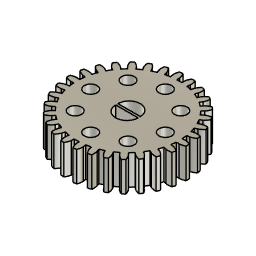
Shaft Arm Joint 0-1 Gear (Autodesk Fusion 360 design; units mm, degrees)
Autodesk Fusion 360 part; units mm, degrees
note: some values were not read from the file. Set by a fixed rule: which sketch regions a step uses.
(part 1 of 20)
sketch "スケッチ1" plane through (0, 0, 0) normal (0, 0, 1) x (1, 0, 0) in component "Component"
  spline S0 degree 5 poles (14.4985, -0.8405) (14.4986, -0.8405) (14.4987, -0.8405) (14.499, -0.8405) (14.4993, -0.8405) (14.4999, -0.8405) (14.5005, -0.8406) (14.5012, -0.8406) (14.502, -0.8406) (14.5028, -0.8406) (14.5037, -0.8407) (14.5048, -0.8407) (14.5058, -0.8407) (14.507, -0.8407) (14.5082, -0.8408) (14.5096, -0.8408) (14.5109, -0.8408) (14.5124, -0.8408) (14.5139, -0.8409) (14.5155, -0.8409) (14.5172, -0.8409) (14.519, -0.8409) (14.5208, -0.8409) (14.5226, -0.8409) (14.5246, -0.8409) (14.5266, -0.8409) (14.5287, -0.8409) (14.5309, -0.8409) (14.5331, -0.8408) (14.5354, -0.8408) (14.5377, -0.8408) (14.5401, -0.8407) (14.5426, -0.8407) (14.5452, -0.8406) (14.5478, -0.8406) (14.5504, -0.8405) (14.5532, -0.8404) (14.556, -0.8403) (14.5588, -0.8402) (14.5617, -0.8401) (14.5647, -0.84) (14.5677, -0.8399) (14.5708, -0.8398) (14.574, -0.8396) (14.5772, -0.8395) (14.5805, -0.8393) (14.5838, -0.8392) (14.5872, -0.839) (14.5906, -0.8388) (14.5941, -0.8386) (14.5977, -0.8384) (14.6013, -0.8382) (14.605, -0.838) (14.6087, -0.8377) (14.6124, -0.8375) (14.6163, -0.8372) (14.6202, -0.8369) (14.6241, -0.8366) (14.6281, -0.8363) (14.6321, -0.836) (14.6362, -0.8357) (14.6404, -0.8354) (14.6446, -0.835) (14.6488, -0.8347) (14.6531, -0.8343) (14.6574, -0.8339) (14.6618, -0.8335) (14.6663, -0.8331) (14.6708, -0.8326) (14.6753, -0.8322) (14.6799, -0.8317) (14.6846, -0.8313) (14.6893, -0.8308) (14.694, -0.8303) (14.6988, -0.8298) (14.7036, -0.8292) (14.7085, -0.8287) (14.7134, -0.8281) (14.7184, -0.8275) (14.7234, -0.8269) (14.7285, -0.8263) (14.7336, -0.8257) (14.7387, -0.8251) (14.7439, -0.8244) (14.7492, -0.8237) (14.7545, -0.8231) (14.7598, -0.8224) (14.7652, -0.8216) (14.7706, -0.8209) (14.7761, -0.8201) (14.7816, -0.8194) (14.7871, -0.8186) (14.7927, -0.8178) (14.7983, -0.817) (14.804, -0.8161) (14.8097, -0.8153) (14.8155, -0.8144) (14.8213, -0.8135) (14.8271, -0.8126) (14.833, -0.8117) (14.8389, -0.8107) (14.8449, -0.8097) (14.8509, -0.8088) (14.8569, -0.8078) (14.863, -0.8067) (14.8691, -0.8057) (14.8753, -0.8047) (14.8814, -0.8036) (14.8877, -0.8025) (14.8939, -0.8014) (14.9003, -0.8002) (14.9066, -0.7991) (14.913, -0.7979) (14.9194, -0.7967) (14.9259, -0.7955) (14.9324, -0.7943) (14.9389, -0.7931) (14.9455, -0.7918) (14.9521, -0.7905) (14.9587, -0.7892) (14.9654, -0.7879) (14.9721, -0.7865) (14.9788, -0.7852) (14.9856, -0.7838) (14.9924, -0.7824) (14.9993, -0.781) (15.0062, -0.7795) (15.0131, -0.778) (15.02, -0.7766) (15.027, -0.775) (15.0341, -0.7735) (15.0411, -0.772) (15.0482, -0.7704) (15.0553, -0.7688) (15.0625, -0.7672) (15.0697, -0.7656) (15.0769, -0.7639) (15.0841, -0.7622) (15.0914, -0.7605) (15.0987, -0.7588) (15.1061, -0.7571) (15.1135, -0.7553) (15.1209, -0.7535) (15.1283, -0.7517) (15.1358, -0.7499) (15.1433, -0.7481) (15.1508, -0.7462) (15.1584, -0.7443) (15.166, -0.7424) (15.1736, -0.7405) (15.1813, -0.7385) (15.1889, -0.7365) (15.1967, -0.7345) (15.2044, -0.7325) (15.2122, -0.7305) (15.22, -0.7284) (15.2278, -0.7263) (15.2357, -0.7242) (15.2436, -0.7221) (15.2515, -0.7199) (15.2594, -0.7177) (15.2674, -0.7155) (15.2754, -0.7133) (15.2834, -0.7111) (15.2915, -0.7088) (15.2996, -0.7065) (15.3077, -0.7042) (15.3158, -0.7018) (15.324, -0.6995) (15.3322, -0.6971) (15.3404, -0.6947) (15.3487, -0.6923) (15.3569, -0.6898) (15.3652, -0.6873) (15.3736, -0.6848) (15.3819, -0.6823) (15.3903, -0.6797) (15.3987, -0.6772) (15.4071, -0.6746) (15.4156, -0.672) (15.4241, -0.6693) (15.4326, -0.6667) (15.4411, -0.664) (15.4497, -0.6613) (15.4582, -0.6585) (15.4668, -0.6558) (15.4755, -0.653) (15.4841, -0.6502) (15.4928, -0.6473) (15.5015, -0.6445) (15.5102, -0.6416) (15.519, -0.6387) (15.5278, -0.6358) (15.5365, -0.6328) (15.5454, -0.6298) (15.5542, -0.6268) (15.5631, -0.6238) (15.572, -0.6207) (15.5809, -0.6177) (15.5898, -0.6146) (15.5988, -0.6114) (15.6077, -0.6083) (15.6167, -0.6051) (15.6258, -0.6019) (15.6348, -0.5987) (15.6439, -0.5955) (15.653, -0.5922) (15.6621, -0.5889) (15.6712, -0.5856) (15.6803, -0.5822) (15.6895, -0.5789) (15.6987, -0.5755) (15.7079, -0.572) (15.7172, -0.5686) (15.7264, -0.5651) (15.7357, -0.5616) (15.745, -0.5581) (15.7543, -0.5546) (15.7636, -0.551) (15.773, -0.5474) (15.7824, -0.5438) (15.7918, -0.5401) (15.8012, -0.5365) (15.8106, -0.5328) (15.8201, -0.529) (15.8295, -0.5253) (15.839, -0.5215) (15.8486, -0.5177) (15.8581, -0.5139) (15.8676, -0.5101) (15.8772, -0.5062) (15.8868, -0.5023) (15.8964, -0.4984) (15.906, -0.4944) (15.9157, -0.4904) (15.9253, -0.4864) (15.935, -0.4824) (15.9447, -0.4784) (15.9544, -0.4743) (15.9641, -0.4702) (15.9739, -0.466) (15.9817, -0.4627) (15.9876, -0.4602) (15.9915, -0.4585) (15.9935, -0.4577) knots 0 0 0 0 0 0 0.00416667 0.00833333 0.0125 0.01666667 0.02083333 0.025 0.02916667 0.03333333 0.0375 0.04166667 0.04583333 0.05 0.05416667 0.05833333 0.0625 0.06666667 0.07083333 0.075 0.07916667 0.08333333 0.0875 0.09166667 0.09583333 0.1 0.10416667 0.10833333 0.1125 0.11666667 0.12083333 0.125 0.12916667 0.13333333 0.1375 0.14166667 0.14583333 0.15 0.15416667 0.15833333 0.1625 0.16666667 0.17083333 0.175 0.17916667 0.18333333 0.1875 0.19166667 0.19583333 0.2 0.20416667 0.20833333 0.2125 0.21666667 0.22083333 0.225 0.22916667 0.23333333 0.2375 0.24166667 0.24583333 0.25 0.25416667 0.25833333 0.2625 0.26666667 0.27083333 0.275 0.27916667 0.28333333 0.2875 0.29166667 0.29583333 0.3 0.30416667 0.30833333 0.3125 0.31666667 0.32083333 0.325 0.32916667 0.33333333 0.3375 0.34166667 0.34583333 0.35 0.35416667 0.35833333 0.3625 0.36666667 0.37083333 0.375 0.37916667 0.38333333 0.3875 0.39166667 0.39583333 0.4 0.40416667 0.40833333 0.4125 0.41666667 0.42083333 0.425 0.42916667 0.43333333 0.4375 0.44166667 0.44583333 0.45 0.45416667 0.45833333 0.4625 0.46666667 0.47083333 0.475 0.47916667 0.48333333 0.4875 0.49166667 0.49583333 0.5 0.50416667 0.50833333 0.5125 0.51666667 0.52083333 0.525 0.52916667 0.53333333 0.5375 0.54166667 0.54583333 0.55 0.55416667 0.55833333 0.5625 0.56666667 0.57083333 0.575 0.57916667 0.58333333 0.5875 0.59166667 0.59583333 0.6 0.60416667 0.60833333 0.6125 0.61666667 0.62083333 0.625 0.62916667 0.63333333 0.6375 0.64166667 0.64583333 0.65 0.65416667 0.65833333 0.6625 0.66666667 0.67083333 0.675 0.67916667 0.68333333 0.6875 0.69166667 0.69583333 0.7 0.70416667 0.70833333 0.7125 0.71666667 0.72083333 0.725 0.72916667 0.73333333 0.7375 0.74166667 0.74583333 0.75 0.75416667 0.75833333 0.7625 0.76666667 0.77083333 0.775 0.77916667 0.78333333 0.7875 0.79166667 0.79583333 0.8 0.80416667 0.80833333 0.8125 0.81666667 0.82083333 0.825 0.82916667 0.83333333 0.8375 0.84166667 0.84583333 0.85 0.85416667 0.85833333 0.8625 0.86666667 0.87083333 0.875 0.87916667 0.88333333 0.8875 0.89166667 0.89583333 0.9 0.90416667 0.90833333 0.9125 0.91666667 0.92083333 0.925 0.92916667 0.93333333 0.9375 0.94166667 0.94583333 0.95 0.95416667 0.95833333 0.9625 0.96666667 0.97083333 0.975 0.97916667 0.98333333 0.9875 0.99166667 0.99583333 1 1 1 1 1 1
  spline S1 degree 5 poles (14.4985, 0.8405) (14.4986, 0.8405) (14.4987, 0.8405) (14.499, 0.8405) (14.4993, 0.8405) (14.4999, 0.8405) (14.5005, 0.8406) (14.5012, 0.8406) (14.502, 0.8406) (14.5028, 0.8406) (14.5037, 0.8407) (14.5048, 0.8407) (14.5058, 0.8407) (14.507, 0.8407) (14.5082, 0.8408) (14.5096, 0.8408) (14.5109, 0.8408) (14.5124, 0.8408) (14.5139, 0.8409) (14.5155, 0.8409) (14.5172, 0.8409) (14.519, 0.8409) (14.5208, 0.8409) (14.5226, 0.8409) (14.5246, 0.8409) (14.5266, 0.8409) (14.5287, 0.8409) (14.5309, 0.8409) (14.5331, 0.8408) (14.5354, 0.8408) (14.5377, 0.8408) (14.5401, 0.8407) (14.5426, 0.8407) (14.5452, 0.8406) (14.5478, 0.8406) (14.5504, 0.8405) (14.5532, 0.8404) (14.556, 0.8403) (14.5588, 0.8402) (14.5617, 0.8401) (14.5647, 0.84) (14.5677, 0.8399) (14.5708, 0.8398) (14.574, 0.8396) (14.5772, 0.8395) (14.5805, 0.8393) (14.5838, 0.8392) (14.5872, 0.839) (14.5906, 0.8388) (14.5941, 0.8386) (14.5977, 0.8384) (14.6013, 0.8382) (14.605, 0.838) (14.6087, 0.8377) (14.6124, 0.8375) (14.6163, 0.8372) (14.6202, 0.8369) (14.6241, 0.8366) (14.6281, 0.8363) (14.6321, 0.836) (14.6362, 0.8357) (14.6404, 0.8354) (14.6446, 0.835) (14.6488, 0.8347) (14.6531, 0.8343) (14.6574, 0.8339) (14.6618, 0.8335) (14.6663, 0.8331) (14.6708, 0.8326) (14.6753, 0.8322) (14.6799, 0.8317) (14.6846, 0.8313) (14.6893, 0.8308) (14.694, 0.8303) (14.6988, 0.8298) (14.7036, 0.8292) (14.7085, 0.8287) (14.7134, 0.8281) (14.7184, 0.8275) (14.7234, 0.8269) (14.7285, 0.8263) (14.7336, 0.8257) (14.7387, 0.8251) (14.7439, 0.8244) (14.7492, 0.8237) (14.7545, 0.8231) (14.7598, 0.8224) (14.7652, 0.8216) (14.7706, 0.8209) (14.7761, 0.8201) (14.7816, 0.8194) (14.7871, 0.8186) (14.7927, 0.8178) (14.7983, 0.817) (14.804, 0.8161) (14.8097, 0.8153) (14.8155, 0.8144) (14.8213, 0.8135) (14.8271, 0.8126) (14.833, 0.8117) (14.8389, 0.8107) (14.8449, 0.8097) (14.8509, 0.8088) (14.8569, 0.8078) (14.863, 0.8067) (14.8691, 0.8057) (14.8753, 0.8047) (14.8814, 0.8036) (14.8877, 0.8025) (14.8939, 0.8014) (14.9003, 0.8002) (14.9066, 0.7991) (14.913, 0.7979) (14.9194, 0.7967) (14.9259, 0.7955) (14.9324, 0.7943) (14.9389, 0.7931) (14.9455, 0.7918) (14.9521, 0.7905) (14.9587, 0.7892) (14.9654, 0.7879) (14.9721, 0.7865) (14.9788, 0.7852) (14.9856, 0.7838) (14.9924, 0.7824) (14.9993, 0.781) (15.0062, 0.7795) (15.0131, 0.778) (15.02, 0.7766) (15.027, 0.775) (15.0341, 0.7735) (15.0411, 0.772) (15.0482, 0.7704) (15.0553, 0.7688) (15.0625, 0.7672) (15.0697, 0.7656) (15.0769, 0.7639) (15.0841, 0.7622) (15.0914, 0.7605) (15.0987, 0.7588) (15.1061, 0.7571) (15.1135, 0.7553) (15.1209, 0.7535) (15.1283, 0.7517) (15.1358, 0.7499) (15.1433, 0.7481) (15.1508, 0.7462) (15.1584, 0.7443) (15.166, 0.7424) (15.1736, 0.7405) (15.1813, 0.7385) (15.1889, 0.7365) (15.1967, 0.7345) (15.2044, 0.7325) (15.2122, 0.7305) (15.22, 0.7284) (15.2278, 0.7263) (15.2357, 0.7242) (15.2436, 0.7221) (15.2515, 0.7199) (15.2594, 0.7177) (15.2674, 0.7155) (15.2754, 0.7133) (15.2834, 0.7111) (15.2915, 0.7088) (15.2996, 0.7065) (15.3077, 0.7042) (15.3158, 0.7018) (15.324, 0.6995) (15.3322, 0.6971) (15.3404, 0.6947) (15.3487, 0.6923) (15.3569, 0.6898) (15.3652, 0.6873) (15.3736, 0.6848) (15.3819, 0.6823) (15.3903, 0.6797) (15.3987, 0.6772) (15.4071, 0.6746) (15.4156, 0.672) (15.4241, 0.6693) (15.4326, 0.6667) (15.4411, 0.664) (15.4497, 0.6613) (15.4582, 0.6585) (15.4668, 0.6558) (15.4755, 0.653) (15.4841, 0.6502) (15.4928, 0.6473) (15.5015, 0.6445) (15.5102, 0.6416) (15.519, 0.6387) (15.5278, 0.6358) (15.5365, 0.6328) (15.5454, 0.6298) (15.5542, 0.6268) (15.5631, 0.6238) (15.572, 0.6207) (15.5809, 0.6177) (15.5898, 0.6146) (15.5988, 0.6114) (15.6077, 0.6083) (15.6167, 0.6051) (15.6258, 0.6019) (15.6348, 0.5987) (15.6439, 0.5955) (15.653, 0.5922) (15.6621, 0.5889) (15.6712, 0.5856) (15.6803, 0.5822) (15.6895, 0.5789) (15.6987, 0.5755) (15.7079, 0.572) (15.7172, 0.5686) (15.7264, 0.5651) (15.7357, 0.5616) (15.745, 0.5581) (15.7543, 0.5546) (15.7636, 0.551) (15.773, 0.5474) (15.7824, 0.5438) (15.7918, 0.5401) (15.8012, 0.5365) (15.8106, 0.5328) (15.8201, 0.529) (15.8295, 0.5253) (15.839, 0.5215) (15.8486, 0.5177) (15.8581, 0.5139) (15.8676, 0.5101) (15.8772, 0.5062) (15.8868, 0.5023) (15.8964, 0.4984) (15.906, 0.4944) (15.9157, 0.4904) (15.9253, 0.4864) (15.935, 0.4824) (15.9447, 0.4784) (15.9544, 0.4743) (15.9641, 0.4702) (15.9739, 0.466) (15.9817, 0.4627) (15.9876, 0.4602) (15.9915, 0.4585) (15.9935, 0.4577) knots 0 0 0 0 0 0 0.00416667 0.00833333 0.0125 0.01666667 0.02083333 0.025 0.02916667 0.03333333 0.0375 0.04166667 0.04583333 0.05 0.05416667 0.05833333 0.0625 0.06666667 0.07083333 0.075 0.07916667 0.08333333 0.0875 0.09166667 0.09583333 0.1 0.10416667 0.10833333 0.1125 0.11666667 0.12083333 0.125 0.12916667 0.13333333 0.1375 0.14166667 0.14583333 0.15 0.15416667 0.15833333 0.1625 0.16666667 0.17083333 0.175 0.17916667 0.18333333 0.1875 0.19166667 0.19583333 0.2 0.20416667 0.20833333 0.2125 0.21666667 0.22083333 0.225 0.22916667 0.23333333 0.2375 0.24166667 0.24583333 0.25 0.25416667 0.25833333 0.2625 0.26666667 0.27083333 0.275 0.27916667 0.28333333 0.2875 0.29166667 0.29583333 0.3 0.30416667 0.30833333 0.3125 0.31666667 0.32083333 0.325 0.32916667 0.33333333 0.3375 0.34166667 0.34583333 0.35 0.35416667 0.35833333 0.3625 0.36666667 0.37083333 0.375 0.37916667 0.38333333 0.3875 0.39166667 0.39583333 0.4 0.40416667 0.40833333 0.4125 0.41666667 0.42083333 0.425 0.42916667 0.43333333 0.4375 0.44166667 0.44583333 0.45 0.45416667 0.45833333 0.4625 0.46666667 0.47083333 0.475 0.47916667 0.48333333 0.4875 0.49166667 0.49583333 0.5 0.50416667 0.50833333 0.5125 0.51666667 0.52083333 0.525 0.52916667 0.53333333 0.5375 0.54166667 0.54583333 0.55 0.55416667 0.55833333 0.5625 0.56666667 0.57083333 0.575 0.57916667 0.58333333 0.5875 0.59166667 0.59583333 0.6 0.60416667 0.60833333 0.6125 0.61666667 0.62083333 0.625 0.62916667 0.63333333 0.6375 0.64166667 0.64583333 0.65 0.65416667 0.65833333 0.6625 0.66666667 0.67083333 0.675 0.67916667 0.68333333 0.6875 0.69166667 0.69583333 0.7 0.70416667 0.70833333 0.7125 0.71666667 0.72083333 0.725 0.72916667 0.73333333 0.7375 0.74166667 0.74583333 0.75 0.75416667 0.75833333 0.7625 0.76666667 0.77083333 0.775 0.77916667 0.78333333 0.7875 0.79166667 0.79583333 0.8 0.80416667 0.80833333 0.8125 0.81666667 0.82083333 0.825 0.82916667 0.83333333 0.8375 0.84166667 0.84583333 0.85 0.85416667 0.85833333 0.8625 0.86666667 0.87083333 0.875 0.87916667 0.88333333 0.8875 0.89166667 0.89583333 0.9 0.90416667 0.90833333 0.9125 0.91666667 0.92083333 0.925 0.92916667 0.93333333 0.9375 0.94166667 0.94583333 0.95 0.95416667 0.95833333 0.9625 0.96666667 0.97083333 0.975 0.97916667 0.98333333 0.9875 0.99166667 0.99583333 1 1 1 1 1 1
  spline S2 degree 5 poles (14.4979, -0.8404) (14.4979, -0.8404) (14.498, -0.8404) (14.498, -0.8404) (14.4981, -0.8404) (14.4983, -0.8405) (14.4984, -0.8405) (14.4984, -0.8405) (14.4985, -0.8405) (14.4985, -0.8405) knots 0 0 0 0 0 0 0.2 0.4 0.6 0.8 1 1 1 1 1 1
  spline S3 degree 5 poles (14.4979, 0.8404) (14.4979, 0.8404) (14.498, 0.8404) (14.498, 0.8404) (14.4981, 0.8404) (14.4983, 0.8405) (14.4984, 0.8405) (14.4984, 0.8405) (14.4985, 0.8405) (14.4985, 0.8405) knots 0 0 0 0 0 0 0.2 0.4 0.6 0.8 1 1 1 1 1 1
  line L0 (0, 0) -> (14.4979, -0.8404)
  line L1 (0, 0) -> (14.4979, 0.8404)
  arc A0 (15.9935, -0.4577) -> (15.9935, 0.4577) centre (0, 0) ccw
  point P0 (14.5005, -0.8406)
  point P1 (14.5037, -0.8407)
  point P2 (14.5082, -0.8408)
  point P3 (14.514, -0.8409)
  point P4 (14.5212, -0.8409)
  point P5 (14.5296, -0.8409)
  point P6 (14.5393, -0.8407)
  point P7 (14.5503, -0.8405)
  point P8 (14.5625, -0.8401)
  point P9 (14.5761, -0.8396)
  point P10 (14.591, -0.8388)
  point P11 (14.6071, -0.8378)
  point P12 (14.6245, -0.8366)
  point P13 (14.6432, -0.8351)
  point P14 (14.6632, -0.8334)
  point P15 (14.6844, -0.8313)
  point P16 (14.707, -0.8288)
  point P17 (14.7307, -0.8261)
  point P18 (14.7557, -0.8229)
  point P19 (14.782, -0.8193)
  point P20 (14.8095, -0.8153)
  point P21 (14.8383, -0.8108)
  point P22 (14.8683, -0.8058)
  point P23 (14.8995, -0.8004)
  point P24 (14.9319, -0.7944)
  point P25 (14.9656, -0.7878)
  point P26 (15.0004, -0.7807)
  point P27 (15.0365, -0.773)
  point P28 (15.0737, -0.7646)
  point P29 (15.1122, -0.7556)
  point P30 (15.1517, -0.746)
  point P31 (15.1925, -0.7356)
  point P32 (15.2344, -0.7245)
  point P33 (15.2774, -0.7127)
  point P34 (15.3216, -0.7002)
  point P35 (15.3669, -0.6868)
  point P36 (15.4133, -0.6727)
  point P37 (15.4608, -0.6577)
  point P38 (15.5094, -0.6419)
  point P39 (15.559, -0.6252)
  point P40 (15.6097, -0.6076)
  point P41 (15.6615, -0.5891)
  point P42 (15.7143, -0.5696)
  point P43 (15.7682, -0.5493)
  point P44 (15.823, -0.5279)
  point P45 (15.8788, -0.5055)
  point P46 (15.9357, -0.4821)
  point P47 (14.5005, 0.8406)
  point P48 (14.5037, 0.8407)
  point P49 (14.5082, 0.8408)
  point P50 (14.514, 0.8409)
  point P51 (14.5212, 0.8409)
  point P52 (14.5296, 0.8409)
  point P53 (14.5393, 0.8407)
  point P54 (14.5503, 0.8405)
  point P55 (14.5625, 0.8401)
  point P56 (14.5761, 0.8396)
  point P57 (14.591, 0.8388)
  point P58 (14.6071, 0.8378)
  point P59 (14.6245, 0.8366)
  point P60 (14.6432, 0.8351)
  point P61 (14.6632, 0.8334)
  point P62 (14.6844, 0.8313)
  point P63 (14.707, 0.8288)
  point P64 (14.7307, 0.8261)
  point P65 (14.7557, 0.8229)
  point P66 (14.782, 0.8193)
  point P67 (14.8095, 0.8153)
  point P68 (14.8383, 0.8108)
  point P69 (14.8683, 0.8058)
  point P70 (14.8995, 0.8004)
  point P71 (14.9319, 0.7944)
  point P72 (14.9656, 0.7878)
  point P73 (15.0004, 0.7807)
  point P74 (15.0365, 0.773)
  point P75 (15.0737, 0.7646)
  point P76 (15.1122, 0.7556)
  point P77 (15.1517, 0.746)
  point P78 (15.1925, 0.7356)
  point P79 (15.2344, 0.7245)
  point P80 (15.2774, 0.7127)
  point P81 (15.3216, 0.7002)
  point P82 (15.3669, 0.6868)
  point P83 (15.4133, 0.6727)
  point P84 (15.4608, 0.6577)
  point P85 (15.5094, 0.6419)
  point P86 (15.559, 0.6252)
  point P87 (15.6097, 0.6076)
  point P88 (15.6615, 0.5891)
  point P89 (15.7143, 0.5696)
  point P90 (15.7682, 0.5493)
  point P91 (15.823, 0.5279)
  point P92 (15.8788, 0.5055)
  point P93 (15.9357, 0.4821)
sketch "スケッチ2" plane through (0, 0, 0) normal (0, 0, 1) x (1, 0, 0) in component "Component"
  circle A0 centre (0, 0) radius 13.75
extrude "押し出し1" add sketch "スケッチ2" along normal blind 8 makes body 1 in component "Component"
extrude "押し出し2" add sketch "スケッチ1" along normal blind 8 separate body makes body 2 in component "Component"
pattern_circular "C パターン1" count 30 over 360 about axis through (0, 0, 1.75) along (0, 0, 1) of "押し出し2" makes body 3 makes body 4 makes body 5 makes body 6 makes body 7 makes body 8 makes body 9 makes body 10 makes body 11 makes body 12 makes body 13 makes body 14 makes body 15 makes body 16 makes body 17 makes body 18 makes body 19 makes body 20 makes body 21 makes body 22 makes body 23 makes body 24 makes body 25 makes body 26 makes body 27 makes body 28 makes body 29 makes body 30 makes body 31 in component "Component"
combine "結合1" operation add target body 1 tool bodies 2 3 4 5 6 7 8 9 10 11 12 13 14 15 16 17 18 19 20 21 22 23 24 25 26 27 28 29 30 31 in component "Component"
sketch "スケッチ3" plane through (0, 0, 0) normal (0, 0, 1) x (1, 0, 0) in component "Component"
  line L0 (0, 0) -> (50.8022, 0) construction
  line L1 (50.8022, 0) -> (50.8022, 3) construction
  line L2 (50.8022, 3) -> (0, 3) construction
  line L3 (0, 3) -> (0, 0) construction
  constraint perpendicular L0 L1
  constraint parallel L0 L2
  constraint parallel L1 L3
sketch "スケッチ1 (2)" plane through (0, 0, 8) normal (0, 0, 1) x (-1, 0, 0)
  arc A0 (-13.5924, 2.0756) -> (-13.727, 0.7957) centre (0, 0) ccw
  line L0 (-13.727, 0.7957) -> (-14.4979, 0.8404)
  line L1 (-14.4979, 0.8404) -> (-14.4985, 0.8405)
  spline S0 degree 5 poles (-14.4985, 0.8405) (-14.4986, 0.8405) (-14.4987, 0.8405) (-14.499, 0.8405) (-14.4993, 0.8405) (-14.4999, 0.8405) (-14.5005, 0.8406) (-14.5012, 0.8406) (-14.502, 0.8406) (-14.5028, 0.8406) (-14.5037, 0.8407) (-14.5048, 0.8407) (-14.5058, 0.8407) (-14.507, 0.8407) (-14.5082, 0.8408) (-14.5096, 0.8408) (-14.5109, 0.8408) (-14.5124, 0.8408) (-14.5139, 0.8409) (-14.5155, 0.8409) (-14.5172, 0.8409) (-14.519, 0.8409) (-14.5208, 0.8409) (-14.5226, 0.8409) (-14.5246, 0.8409) (-14.5266, 0.8409) (-14.5287, 0.8409) (-14.5309, 0.8409) (-14.5331, 0.8408) (-14.5354, 0.8408) (-14.5377, 0.8408) (-14.5401, 0.8407) (-14.5426, 0.8407) (-14.5452, 0.8406) (-14.5478, 0.8406) (-14.5504, 0.8405) (-14.5532, 0.8404) (-14.556, 0.8403) (-14.5588, 0.8402) (-14.5617, 0.8401) (-14.5647, 0.84) (-14.5677, 0.8399) (-14.5708, 0.8398) (-14.574, 0.8396) (-14.5772, 0.8395) (-14.5805, 0.8393) (-14.5838, 0.8392) (-14.5872, 0.839) (-14.5906, 0.8388) (-14.5941, 0.8386) (-14.5977, 0.8384) (-14.6013, 0.8382) (-14.605, 0.838) (-14.6087, 0.8377) (-14.6124, 0.8375) (-14.6163, 0.8372) (-14.6202, 0.8369) (-14.6241, 0.8366) (-14.6281, 0.8363) (-14.6321, 0.836) (-14.6362, 0.8357) (-14.6404, 0.8354) (-14.6446, 0.835) (-14.6488, 0.8347) (-14.6531, 0.8343) (-14.6574, 0.8339) (-14.6618, 0.8335) (-14.6663, 0.8331) (-14.6708, 0.8326) (-14.6753, 0.8322) (-14.6799, 0.8317) (-14.6846, 0.8313) (-14.6893, 0.8308) (-14.694, 0.8303) (-14.6988, 0.8298) (-14.7036, 0.8292) (-14.7085, 0.8287) (-14.7134, 0.8281) (-14.7184, 0.8275) (-14.7234, 0.8269) (-14.7285, 0.8263) (-14.7336, 0.8257) (-14.7387, 0.8251) (-14.7439, 0.8244) (-14.7492, 0.8237) (-14.7545, 0.8231) (-14.7598, 0.8224) (-14.7652, 0.8216) (-14.7706, 0.8209) (-14.7761, 0.8201) (-14.7816, 0.8194) (-14.7871, 0.8186) (-14.7927, 0.8178) (-14.7983, 0.817) (-14.804, 0.8161) (-14.8097, 0.8153) (-14.8155, 0.8144) (-14.8213, 0.8135) (-14.8271, 0.8126) (-14.833, 0.8117) (-14.8389, 0.8107) (-14.8449, 0.8097) (-14.8509, 0.8088) (-14.8569, 0.8078) (-14.863, 0.8067) (-14.8691, 0.8057) (-14.8753, 0.8047) (-14.8814, 0.8036) (-14.8877, 0.8025) (-14.8939, 0.8014) (-14.9003, 0.8002) (-14.9066, 0.7991) (-14.913, 0.7979) (-14.9194, 0.7967) (-14.9259, 0.7955) (-14.9324, 0.7943) (-14.9389, 0.7931) (-14.9455, 0.7918) (-14.9521, 0.7905) (-14.9587, 0.7892) (-14.9654, 0.7879) (-14.9721, 0.7865) (-14.9788, 0.7852) (-14.9856, 0.7838) (-14.9924, 0.7824) (-14.9993, 0.781) (-15.0062, 0.7795) (-15.0131, 0.778) (-15.02, 0.7766) (-15.027, 0.775) (-15.0341, 0.7735) (-15.0411, 0.772) (-15.0482, 0.7704) (-15.0553, 0.7688) (-15.0625, 0.7672) (-15.0697, 0.7656) (-15.0769, 0.7639) (-15.0841, 0.7622) (-15.0914, 0.7605) (-15.0987, 0.7588) (-15.1061, 0.7571) (-15.1135, 0.7553) (-15.1209, 0.7535) (-15.1283, 0.7517) (-15.1358, 0.7499) (-15.1433, 0.7481) (-15.1508, 0.7462) (-15.1584, 0.7443) (-15.166, 0.7424) (-15.1736, 0.7405) (-15.1813, 0.7385) (-15.1889, 0.7365) (-15.1967, 0.7345) (-15.2044, 0.7325) (-15.2122, 0.7305) (-15.22, 0.7284) (-15.2278, 0.7263) (-15.2357, 0.7242) (-15.2436, 0.7221) (-15.2515, 0.7199) (-15.2594, 0.7177) (-15.2674, 0.7155) (-15.2754, 0.7133) (-15.2834, 0.7111) (-15.2915, 0.7088) (-15.2996, 0.7065) (-15.3077, 0.7042) (-15.3158, 0.7018) (-15.324, 0.6995) (-15.3322, 0.6971) (-15.3404, 0.6947) (-15.3487, 0.6923) (-15.3569, 0.6898) (-15.3652, 0.6873) (-15.3736, 0.6848) (-15.3819, 0.6823) (-15.3903, 0.6797) (-15.3987, 0.6772) (-15.4071, 0.6746) (-15.4156, 0.672) (-15.4241, 0.6693) (-15.4326, 0.6667) (-15.4411, 0.664) (-15.4497, 0.6613) (-15.4582, 0.6585) (-15.4668, 0.6558) (-15.4755, 0.653) (-15.4841, 0.6502) (-15.4928, 0.6473) (-15.5015, 0.6445) (-15.5102, 0.6416) (-15.519, 0.6387) (-15.5278, 0.6358) (-15.5365, 0.6328) (-15.5454, 0.6298) (-15.5542, 0.6268) (-15.5631, 0.6238) (-15.572, 0.6207) (-15.5809, 0.6177) (-15.5898, 0.6146) (-15.5988, 0.6114) (-15.6077, 0.6083) (-15.6167, 0.6051) (-15.6258, 0.6019) (-15.6348, 0.5987) (-15.6439, 0.5955) (-15.653, 0.5922) (-15.6621, 0.5889) (-15.6712, 0.5856) (-15.6803, 0.5822) (-15.6895, 0.5789) (-15.6987, 0.5755) (-15.7079, 0.572) (-15.7172, 0.5686) (-15.7264, 0.5651) (-15.7357, 0.5616) (-15.745, 0.5581) (-15.7543, 0.5546) (-15.7636, 0.551) (-15.773, 0.5474) (-15.7824, 0.5438) (-15.7918, 0.5401) (-15.8012, 0.5365) (-15.8106, 0.5328) (-15.8201, 0.529) (-15.8295, 0.5253) (-15.839, 0.5215) (-15.8486, 0.5177) (-15.8581, 0.5139) (-15.8676, 0.5101) (-15.8772, 0.5062) (-15.8868, 0.5023) (-15.8964, 0.4984) (-15.906, 0.4944) (-15.9157, 0.4904) (-15.9253, 0.4864) (-15.935, 0.4824) (-15.9447, 0.4784) (-15.9544, 0.4743) (-15.9641, 0.4702) (-15.9739, 0.466) (-15.9817, 0.4627) (-15.9876, 0.4602) (-15.9915, 0.4585) (-15.9935, 0.4577) knots 0 0 0 0 0 0 0.00416667 0.00833333 0.0125 0.01666667 0.02083333 0.025 0.02916667 0.03333333 0.0375 0.04166667 0.04583333 0.05 0.05416667 0.05833333 0.0625 0.06666667 0.07083333 0.075 0.07916667 0.08333333 0.0875 0.09166667 0.09583333 0.1 0.10416667 0.10833333 0.1125 0.11666667 0.12083333 0.125 0.12916667 0.13333333 0.1375 0.14166667 0.14583333 0.15 0.15416667 0.15833333 0.1625 0.16666667 0.17083333 0.175 0.17916667 0.18333333 0.1875 0.19166667 0.19583333 0.2 0.20416667 0.20833333 0.2125 0.21666667 0.22083333 0.225 0.22916667 0.23333333 0.2375 0.24166667 0.24583333 0.25 0.25416667 0.25833333 0.2625 0.26666667 0.27083333 0.275 0.27916667 0.28333333 0.2875 0.29166667 0.29583333 0.3 0.30416667 0.30833333 0.3125 0.31666667 0.32083333 0.325 0.32916667 0.33333333 0.3375 0.34166667 0.34583333 0.35 0.35416667 0.35833333 0.3625 0.36666667 0.37083333 0.375 0.37916667 0.38333333 0.3875 0.39166667 0.39583333 0.4 0.40416667 0.40833333 0.4125 0.41666667 0.42083333 0.425 0.42916667 0.43333333 0.4375 0.44166667 0.44583333 0.45 0.45416667 0.45833333 0.4625 0.46666667 0.47083333 0.475 0.47916667 0.48333333 0.4875 0.49166667 0.49583333 0.5 0.50416667 0.50833333 0.5125 0.51666667 0.52083333 0.525 0.52916667 0.53333333 0.5375 0.54166667 0.54583333 0.55 0.55416667 0.55833333 0.5625 0.56666667 0.57083333 0.575 0.57916667 0.58333333 0.5875 0.59166667 0.59583333 0.6 0.60416667 0.60833333 0.6125 0.61666667 0.62083333 0.625 0.62916667 0.63333333 0.6375 0.64166667 0.64583333 0.65 0.65416667 0.65833333 0.6625 0.66666667 0.67083333 0.675 0.67916667 0.68333333 0.6875 0.69166667 0.69583333 0.7 0.70416667 0.70833333 0.7125 0.71666667 0.72083333 0.725 0.72916667 0.73333333 0.7375 0.74166667 0.74583333 0.75 0.75416667 0.75833333 0.7625 0.76666667 0.77083333 0.775 0.77916667 0.78333333 0.7875 0.79166667 0.79583333 0.8 0.80416667 0.80833333 0.8125 0.81666667 0.82083333 0.825 0.82916667 0.83333333 0.8375 0.84166667 0.84583333 0.85 0.85416667 0.85833333 0.8625 0.86666667 0.87083333 0.875 0.87916667 0.88333333 0.8875 0.89166667 0.89583333 0.9 0.90416667 0.90833333 0.9125 0.91666667 0.92083333 0.925 0.92916667 0.93333333 0.9375 0.94166667 0.94583333 0.95 0.95416667 0.95833333 0.9625 0.96666667 0.97083333 0.975 0.97916667 0.98333333 0.9875 0.99166667 0.99583333 1 1 1 1 1 1
  arc A1 (-15.9935, 0.4577) -> (-15.9935, -0.4577) centre (0, 0) ccw
  spline S1 degree 5 poles (-15.9935, -0.4577) (-15.9915, -0.4585) (-15.9876, -0.4602) (-15.9817, -0.4627) (-15.9739, -0.466) (-15.9641, -0.4702) (-15.9544, -0.4743) (-15.9447, -0.4784) (-15.935, -0.4824) (-15.9253, -0.4864) (-15.9157, -0.4904) (-15.906, -0.4944) (-15.8964, -0.4984) (-15.8868, -0.5023) (-15.8772, -0.5062) (-15.8676, -0.5101) (-15.8581, -0.5139) (-15.8486, -0.5177) (-15.839, -0.5215) (-15.8295, -0.5253) (-15.8201, -0.529) (-15.8106, -0.5328) (-15.8012, -0.5365) (-15.7918, -0.5401) (-15.7824, -0.5438) (-15.773, -0.5474) (-15.7636, -0.551) (-15.7543, -0.5546) (-15.745, -0.5581) (-15.7357, -0.5616) (-15.7264, -0.5651) (-15.7172, -0.5686) (-15.7079, -0.572) (-15.6987, -0.5755) (-15.6895, -0.5789) (-15.6803, -0.5822) (-15.6712, -0.5856) (-15.6621, -0.5889) (-15.653, -0.5922) (-15.6439, -0.5955) (-15.6348, -0.5987) (-15.6258, -0.6019) (-15.6167, -0.6051) (-15.6077, -0.6083) (-15.5988, -0.6114) (-15.5898, -0.6146) (-15.5809, -0.6177) (-15.572, -0.6207) (-15.5631, -0.6238) (-15.5542, -0.6268) (-15.5454, -0.6298) (-15.5365, -0.6328) (-15.5278, -0.6358) (-15.519, -0.6387) (-15.5102, -0.6416) (-15.5015, -0.6445) (-15.4928, -0.6473) (-15.4841, -0.6502) (-15.4755, -0.653) (-15.4668, -0.6558) (-15.4582, -0.6585) (-15.4497, -0.6613) (-15.4411, -0.664) (-15.4326, -0.6667) (-15.4241, -0.6693) (-15.4156, -0.672) (-15.4071, -0.6746) (-15.3987, -0.6772) (-15.3903, -0.6797) (-15.3819, -0.6823) (-15.3736, -0.6848) (-15.3652, -0.6873) (-15.3569, -0.6898) (-15.3487, -0.6923) (-15.3404, -0.6947) (-15.3322, -0.6971) (-15.324, -0.6995) (-15.3158, -0.7018) (-15.3077, -0.7042) (-15.2996, -0.7065) (-15.2915, -0.7088) (-15.2834, -0.7111) (-15.2754, -0.7133) (-15.2674, -0.7155) (-15.2594, -0.7177) (-15.2515, -0.7199) (-15.2436, -0.7221) (-15.2357, -0.7242) (-15.2278, -0.7263) (-15.22, -0.7284) (-15.2122, -0.7305) (-15.2044, -0.7325) (-15.1967, -0.7345) (-15.1889, -0.7365) (-15.1813, -0.7385) (-15.1736, -0.7405) (-15.166, -0.7424) (-15.1584, -0.7443) (-15.1508, -0.7462) (-15.1433, -0.7481) (-15.1358, -0.7499) (-15.1283, -0.7517) (-15.1209, -0.7535) (-15.1135, -0.7553) (-15.1061, -0.7571) (-15.0987, -0.7588) (-15.0914, -0.7605) (-15.0841, -0.7622) (-15.0769, -0.7639) (-15.0697, -0.7656) (-15.0625, -0.7672) (-15.0553, -0.7688) (-15.0482, -0.7704) (-15.0411, -0.772) (-15.0341, -0.7735) (-15.027, -0.775) (-15.02, -0.7766) (-15.0131, -0.778) (-15.0062, -0.7795) (-14.9993, -0.781) (-14.9924, -0.7824) (-14.9856, -0.7838) (-14.9788, -0.7852) (-14.9721, -0.7865) (-14.9654, -0.7879) (-14.9587, -0.7892) (-14.9521, -0.7905) (-14.9455, -0.7918) (-14.9389, -0.7931) (-14.9324, -0.7943) (-14.9259, -0.7955) (-14.9194, -0.7967) (-14.913, -0.7979) (-14.9066, -0.7991) (-14.9003, -0.8002) (-14.8939, -0.8014) (-14.8877, -0.8025) (-14.8814, -0.8036) (-14.8753, -0.8047) (-14.8691, -0.8057) (-14.863, -0.8067) (-14.8569, -0.8078) (-14.8509, -0.8088) (-14.8449, -0.8097) (-14.8389, -0.8107) (-14.833, -0.8117) (-14.8271, -0.8126) (-14.8213, -0.8135) (-14.8155, -0.8144) (-14.8097, -0.8153) (-14.804, -0.8161) (-14.7983, -0.817) (-14.7927, -0.8178) (-14.7871, -0.8186) (-14.7816, -0.8194) (-14.7761, -0.8201) (-14.7706, -0.8209) (-14.7652, -0.8216) (-14.7598, -0.8224) (-14.7545, -0.8231) (-14.7492, -0.8237) (-14.7439, -0.8244) (-14.7387, -0.8251) (-14.7336, -0.8257) (-14.7285, -0.8263) (-14.7234, -0.8269) (-14.7184, -0.8275) (-14.7134, -0.8281) (-14.7085, -0.8287) (-14.7036, -0.8292) (-14.6988, -0.8298) (-14.694, -0.8303) (-14.6893, -0.8308) (-14.6846, -0.8313) (-14.6799, -0.8317) (-14.6753, -0.8322) (-14.6708, -0.8326) (-14.6663, -0.8331) (-14.6618, -0.8335) (-14.6574, -0.8339) (-14.6531, -0.8343) (-14.6488, -0.8347) (-14.6446, -0.835) (-14.6404, -0.8354) (-14.6362, -0.8357) (-14.6321, -0.836) (-14.6281, -0.8363) (-14.6241, -0.8366) (-14.6202, -0.8369) (-14.6163, -0.8372) (-14.6124, -0.8375) (-14.6087, -0.8377) (-14.605, -0.838) (-14.6013, -0.8382) (-14.5977, -0.8384) (-14.5941, -0.8386) (-14.5906, -0.8388) (-14.5872, -0.839) (-14.5838, -0.8392) (-14.5805, -0.8393) (-14.5772, -0.8395) (-14.574, -0.8396) (-14.5708, -0.8398) (-14.5677, -0.8399) (-14.5647, -0.84) (-14.5617, -0.8401) (-14.5588, -0.8402) (-14.556, -0.8403) (-14.5532, -0.8404) (-14.5504, -0.8405) (-14.5478, -0.8406) (-14.5452, -0.8406) (-14.5426, -0.8407) (-14.5401, -0.8407) (-14.5377, -0.8408) (-14.5354, -0.8408) (-14.5331, -0.8408) (-14.5309, -0.8409) (-14.5287, -0.8409) (-14.5266, -0.8409) (-14.5246, -0.8409) (-14.5226, -0.8409) (-14.5208, -0.8409) (-14.519, -0.8409) (-14.5172, -0.8409) (-14.5155, -0.8409) (-14.5139, -0.8409) (-14.5124, -0.8408) (-14.5109, -0.8408) (-14.5096, -0.8408) (-14.5082, -0.8408) (-14.507, -0.8407) (-14.5058, -0.8407) (-14.5048, -0.8407) (-14.5037, -0.8407) (-14.5028, -0.8406) (-14.502, -0.8406) (-14.5012, -0.8406) (-14.5005, -0.8406) (-14.4999, -0.8405) (-14.4993, -0.8405) (-14.499, -0.8405) (-14.4987, -0.8405) (-14.4986, -0.8405) (-14.4985, -0.8405) knots -1 -1 -1 -1 -1 -1 -0.99583333 -0.99166667 -0.9875 -0.98333333 -0.97916667 -0.975 -0.97083333 -0.96666667 -0.9625 -0.95833333 -0.95416667 -0.95 -0.94583333 -0.94166667 -0.9375 -0.93333333 -0.92916667 -0.925 -0.92083333 -0.91666667 -0.9125 -0.90833333 -0.90416667 -0.9 -0.89583333 -0.89166667 -0.8875 -0.88333333 -0.87916667 -0.875 -0.87083333 -0.86666667 -0.8625 -0.85833333 -0.85416667 -0.85 -0.84583333 -0.84166667 -0.8375 -0.83333333 -0.82916667 -0.825 -0.82083333 -0.81666667 -0.8125 -0.80833333 -0.80416667 -0.8 -0.79583333 -0.79166667 -0.7875 -0.78333333 -0.77916667 -0.775 -0.77083333 -0.76666667 -0.7625 -0.75833333 -0.75416667 -0.75 -0.74583333 -0.74166667 -0.7375 -0.73333333 -0.72916667 -0.725 -0.72083333 -0.71666667 -0.7125 -0.70833333 -0.70416667 -0.7 -0.69583333 -0.69166667 -0.6875 -0.68333333 -0.67916667 -0.675 -0.67083333 -0.66666667 -0.6625 -0.65833333 -0.65416667 -0.65 -0.64583333 -0.64166667 -0.6375 -0.63333333 -0.62916667 -0.625 -0.62083333 -0.61666667 -0.6125 -0.60833333 -0.60416667 -0.6 -0.59583333 -0.59166667 -0.5875 -0.58333333 -0.57916667 -0.575 -0.57083333 -0.56666667 -0.5625 -0.55833333 -0.55416667 -0.55 -0.54583333 -0.54166667 -0.5375 -0.53333333 -0.52916667 -0.525 -0.52083333 -0.51666667 -0.5125 -0.50833333 -0.50416667 -0.5 -0.49583333 -0.49166667 -0.4875 -0.48333333 -0.47916667 -0.475 -0.47083333 -0.46666667 -0.4625 -0.45833333 -0.45416667 -0.45 -0.44583333 -0.44166667 -0.4375 -0.43333333 -0.42916667 -0.425 -0.42083333 -0.41666667 -0.4125 -0.40833333 -0.40416667 -0.4 -0.39583333 -0.39166667 -0.3875 -0.38333333 -0.37916667 -0.375 -0.37083333 -0.36666667 -0.3625 -0.35833333 -0.35416667 -0.35 -0.34583333 -0.34166667 -0.3375 -0.33333333 -0.32916667 -0.325 -0.32083333 -0.31666667 -0.3125 -0.30833333 -0.30416667 -0.3 -0.29583333 -0.29166667 -0.2875 -0.28333333 -0.27916667 -0.275 -0.27083333 -0.26666667 -0.2625 -0.25833333 -0.25416667 -0.25 -0.24583333 -0.24166667 -0.2375 -0.23333333 -0.22916667 -0.225 -0.22083333 -0.21666667 -0.2125 -0.20833333 -0.20416667 -0.2 -0.19583333 -0.19166667 -0.1875 -0.18333333 -0.17916667 -0.175 -0.17083333 -0.16666667 -0.1625 -0.15833333 -0.15416667 -0.15 -0.14583333 -0.14166667 -0.1375 -0.13333333 -0.12916667 -0.125 -0.12083333 -0.11666667 -0.1125 -0.10833333 -0.10416667 -0.1 -0.09583333 -0.09166667 -0.0875 -0.08333333 -0.07916667 -0.075 -0.07083333 -0.06666667 -0.0625 -0.05833333 -0.05416667 -0.05 -0.04583333 -0.04166667 -0.0375 -0.03333333 -0.02916667 -0.025 -0.02083333 -0.01666667 -0.0125 -0.00833333 -0.00416667 0 0 0 0 0 0
  line L2 (-14.4985, -0.8405) -> (-14.4979, -0.8404)
  line L3 (-14.4979, -0.8404) -> (-13.727, -0.7957)
  arc A2 (-13.727, -0.7957) -> (-13.5924, -2.0756) centre (0, 0) ccw
  line L4 (-13.5924, -2.0756) -> (-14.3558, -2.1922)
  line L5 (-14.3558, -2.1922) -> (-14.3564, -2.1923)
  spline S2 degree 5 poles (-14.3564, -2.1923) (-14.3565, -2.1923) (-14.3566, -2.1923) (-14.3569, -2.1924) (-14.3572, -2.1924) (-14.3578, -2.1925) (-14.3584, -2.1926) (-14.3591, -2.1928) (-14.3598, -2.1929) (-14.3607, -2.193) (-14.3616, -2.1932) (-14.3626, -2.1934) (-14.3637, -2.1936) (-14.3648, -2.1938) (-14.366, -2.194) (-14.3673, -2.1943) (-14.3687, -2.1945) (-14.3701, -2.1948) (-14.3716, -2.1951) (-14.3732, -2.1954) (-14.3748, -2.1958) (-14.3765, -2.1961) (-14.3783, -2.1965) (-14.3801, -2.1969) (-14.382, -2.1973) (-14.384, -2.1977) (-14.386, -2.1982) (-14.3882, -2.1986) (-14.3903, -2.1991) (-14.3925, -2.1996) (-14.3948, -2.2002) (-14.3972, -2.2007) (-14.3996, -2.2013) (-14.4021, -2.2018) (-14.4046, -2.2025) (-14.4072, -2.2031) (-14.4099, -2.2037) (-14.4126, -2.2044) (-14.4154, -2.2051) (-14.4182, -2.2058) (-14.4211, -2.2065) (-14.424, -2.2072) (-14.427, -2.208) (-14.4301, -2.2088) (-14.4332, -2.2096) (-14.4364, -2.2104) (-14.4396, -2.2113) (-14.4429, -2.2122) (-14.4462, -2.2131) (-14.4496, -2.214) (-14.453, -2.2149) (-14.4565, -2.2159) (-14.46, -2.2169) (-14.4636, -2.2179) (-14.4673, -2.2189) (-14.4709, -2.22) (-14.4747, -2.2211) (-14.4785, -2.2222) (-14.4823, -2.2233) (-14.4862, -2.2244) (-14.4901, -2.2256) (-14.4941, -2.2268) (-14.4981, -2.228) (-14.5022, -2.2292) (-14.5063, -2.2305) (-14.5105, -2.2318) (-14.5147, -2.2331) (-14.519, -2.2344) (-14.5233, -2.2358) (-14.5277, -2.2372) (-14.5321, -2.2386) (-14.5365, -2.24) (-14.541, -2.2414) (-14.5455, -2.2429) (-14.5501, -2.2444) (-14.5547, -2.2459) (-14.5594, -2.2475) (-14.5641, -2.2491) (-14.5688, -2.2507) (-14.5736, -2.2523) (-14.5784, -2.2539) (-14.5833, -2.2556) (-14.5882, -2.2573) (-14.5932, -2.259) (-14.5981, -2.2608) (-14.6032, -2.2626) (-14.6082, -2.2644) (-14.6133, -2.2662) (-14.6185, -2.268) (-14.6237, -2.2699) (-14.6289, -2.2718) (-14.6342, -2.2737) (-14.6395, -2.2757) (-14.6448, -2.2776) (-14.6502, -2.2796) (-14.6556, -2.2817) (-14.661, -2.2837) (-14.6665, -2.2858) (-14.672, -2.2879) (-14.6776, -2.29) (-14.6832, -2.2922) (-14.6888, -2.2944) (-14.6945, -2.2966) (-14.7002, -2.2988) (-14.7059, -2.3011) (-14.7117, -2.3034) (-14.7175, -2.3057) (-14.7233, -2.308) (-14.7292, -2.3104) (-14.7351, -2.3128) (-14.741, -2.3152) (-14.747, -2.3176) (-14.753, -2.3201) (-14.759, -2.3226) (-14.7651, -2.3251) (-14.7712, -2.3277) (-14.7773, -2.3302) (-14.7835, -2.3328) (-14.7897, -2.3355) (-14.7959, -2.3381) (-14.8022, -2.3408) (-14.8084, -2.3435) (-14.8148, -2.3463) (-14.8211, -2.349) (-14.8275, -2.3518) (-14.8339, -2.3546) (-14.8403, -2.3575) (-14.8468, -2.3604) (-14.8533, -2.3633) (-14.8598, -2.3662) (-14.8663, -2.3691) (-14.8729, -2.3721) (-14.8795, -2.3751) (-14.8862, -2.3782) (-14.8928, -2.3812) (-14.8995, -2.3843) (-14.9062, -2.3874) (-14.913, -2.3906) (-14.9198, -2.3938) (-14.9266, -2.397) (-14.9334, -2.4002) (-14.9402, -2.4034) (-14.9471, -2.4067) (-14.954, -2.41) (-14.9609, -2.4134) (-14.9679, -2.4167) (-14.9749, -2.4201) (-14.9819, -2.4236) (-14.9889, -2.427) (-14.996, -2.4305) (-15.0031, -2.434) (-15.0102, -2.4375) (-15.0173, -2.4411) (-15.0245, -2.4447) (-15.0316, -2.4483) (-15.0388, -2.4519) (-15.0461, -2.4556) (-15.0533, -2.4593) (-15.0606, -2.463) (-15.0679, -2.4668) (-15.0752, -2.4706) (-15.0825, -2.4744) (-15.0899, -2.4782) (-15.0973, -2.4821) (-15.1047, -2.486) (-15.1121, -2.4899) (-15.1196, -2.4939) (-15.1271, -2.4978) (-15.1346, -2.5018) (-15.1421, -2.5059) (-15.1496, -2.5099) (-15.1572, -2.514) (-15.1648, -2.5182) (-15.1724, -2.5223) (-15.18, -2.5265) (-15.1876, -2.5307) (-15.1953, -2.5349) (-15.203, -2.5392) (-15.2107, -2.5435) (-15.2184, -2.5478) (-15.2262, -2.5522) (-15.2339, -2.5565) (-15.2417, -2.5609) (-15.2495, -2.5654) (-15.2574, -2.5698) (-15.2652, -2.5743) (-15.2731, -2.5788) (-15.2809, -2.5834) (-15.2888, -2.588) (-15.2968, -2.5926) (-15.3047, -2.5972) (-15.3126, -2.6019) (-15.3206, -2.6065) (-15.3286, -2.6113) (-15.3366, -2.616) (-15.3446, -2.6208) (-15.3527, -2.6256) (-15.3607, -2.6304) (-15.3688, -2.6353) (-15.3769, -2.6402) (-15.385, -2.6451) (-15.3931, -2.65) (-15.4013, -2.655) (-15.4094, -2.66) (-15.4176, -2.665) (-15.4258, -2.6701) (-15.434, -2.6752) (-15.4422, -2.6803) (-15.4505, -2.6855) (-15.4587, -2.6906) (-15.467, -2.6958) (-15.4753, -2.7011) (-15.4836, -2.7063) (-15.4919, -2.7116) (-15.5002, -2.7169) (-15.5086, -2.7223) (-15.517, -2.7277) (-15.5253, -2.7331) (-15.5337, -2.7385) (-15.5421, -2.744) (-15.5505, -2.7494) (-15.559, -2.755) (-15.5674, -2.7605) (-15.5759, -2.7661) (-15.5844, -2.7717) (-15.5929, -2.7773) (-15.6014, -2.783) (-15.6099, -2.7887) (-15.6184, -2.7944) (-15.6269, -2.8002) (-15.6355, -2.8059) (-15.6441, -2.8117) (-15.6526, -2.8176) (-15.6612, -2.8234) (-15.6698, -2.8293) (-15.6785, -2.8353) (-15.6871, -2.8412) (-15.6957, -2.8472) (-15.7044, -2.8532) (-15.713, -2.8592) (-15.7217, -2.8653) (-15.7287, -2.8702) (-15.7339, -2.8738) (-15.7374, -2.8763) (-15.7391, -2.8775) knots 0 0 0 0 0 0 0.00416667 0.00833333 0.0125 0.01666667 0.02083333 0.025 0.02916667 0.03333333 0.0375 0.04166667 0.04583333 0.05 0.05416667 0.05833333 0.0625 0.06666667 0.07083333 0.075 0.07916667 0.08333333 0.0875 0.09166667 0.09583333 0.1 0.10416667 0.10833333 0.1125 0.11666667 0.12083333 0.125 0.12916667 0.13333333 0.1375 0.14166667 0.14583333 0.15 0.15416667 0.15833333 0.1625 0.16666667 0.17083333 0.175 0.17916667 0.18333333 0.1875 0.19166667 0.19583333 0.2 0.20416667 0.20833333 0.2125 0.21666667 0.22083333 0.225 0.22916667 0.23333333 0.2375 0.24166667 0.24583333 0.25 0.25416667 0.25833333 0.2625 0.26666667 0.27083333 0.275 0.27916667 0.28333333 0.2875 0.29166667 0.29583333 0.3 0.30416667 0.30833333 0.3125 0.31666667 0.32083333 0.325 0.32916667 0.33333333 0.3375 0.34166667 0.34583333 0.35 0.35416667 0.35833333 0.3625 0.36666667 0.37083333 0.375 0.37916667 0.38333333 0.3875 0.39166667 0.39583333 0.4 0.40416667 0.40833333 0.4125 0.41666667 0.42083333 0.425 0.42916667 0.43333333 0.4375 0.44166667 0.44583333 0.45 0.45416667 0.45833333 0.4625 0.46666667 0.47083333 0.475 0.47916667 0.48333333 0.4875 0.49166667 0.49583333 0.5 0.50416667 0.50833333 0.5125 0.51666667 0.52083333 0.525 0.52916667 0.53333333 0.5375 0.54166667 0.54583333 0.55 0.55416667 0.55833333 0.5625 0.56666667 0.57083333 0.575 0.57916667 0.58333333 0.5875 0.59166667 0.59583333 0.6 0.60416667 0.60833333 0.6125 0.61666667 0.62083333 0.625 0.62916667 0.63333333 0.6375 0.64166667 0.64583333 0.65 0.65416667 0.65833333 0.6625 0.66666667 0.67083333 0.675 0.67916667 0.68333333 0.6875 0.69166667 0.69583333 0.7 0.70416667 0.70833333 0.7125 0.71666667 0.72083333 0.725 0.72916667 0.73333333 0.7375 0.74166667 0.74583333 0.75 0.75416667 0.75833333 0.7625 0.76666667 0.77083333 0.775 0.77916667 0.78333333 0.7875 0.79166667 0.79583333 0.8 0.80416667 0.80833333 0.8125 0.81666667 0.82083333 0.825 0.82916667 0.83333333 0.8375 0.84166667 0.84583333 0.85 0.85416667 0.85833333 0.8625 0.86666667 0.87083333 0.875 0.87916667 0.88333333 0.8875 0.89166667 0.89583333 0.9 0.90416667 0.90833333 0.9125 0.91666667 0.92083333 0.925 0.92916667 0.93333333 0.9375 0.94166667 0.94583333 0.95 0.95416667 0.95833333 0.9625 0.96666667 0.97083333 0.975 0.97916667 0.98333333 0.9875 0.99166667 0.99583333 1 1 1 1 1 1
  arc A3 (-15.7391, -2.8775) -> (-15.5488, -3.7729) centre (0, 0) ccw
  spline S3 degree 5 poles (-15.5488, -3.7729) (-15.5467, -3.7733) (-15.5425, -3.7742) (-15.5363, -3.7754) (-15.5279, -3.777) (-15.5175, -3.779) (-15.5072, -3.781) (-15.4968, -3.783) (-15.4865, -3.7849) (-15.4762, -3.7869) (-15.4659, -3.7888) (-15.4556, -3.7907) (-15.4454, -3.7925) (-15.4352, -3.7944) (-15.425, -3.7962) (-15.4148, -3.798) (-15.4047, -3.7998) (-15.3946, -3.8015) (-15.3845, -3.8033) (-15.3744, -3.805) (-15.3644, -3.8067) (-15.3544, -3.8083) (-15.3444, -3.81) (-15.3344, -3.8116) (-15.3244, -3.8132) (-15.3145, -3.8148) (-15.3046, -3.8164) (-15.2947, -3.8179) (-15.2849, -3.8195) (-15.2751, -3.821) (-15.2653, -3.8225) (-15.2555, -3.8239) (-15.2457, -3.8254) (-15.236, -3.8268) (-15.2263, -3.8282) (-15.2166, -3.8296) (-15.207, -3.831) (-15.1974, -3.8323) (-15.1878, -3.8337) (-15.1782, -3.835) (-15.1687, -3.8363) (-15.1591, -3.8375) (-15.1497, -3.8388) (-15.1402, -3.84) (-15.1308, -3.8412) (-15.1214, -3.8424) (-15.112, -3.8436) (-15.1026, -3.8448) (-15.0933, -3.8459) (-15.084, -3.847) (-15.0747, -3.8481) (-15.0655, -3.8492) (-15.0563, -3.8503) (-15.0471, -3.8513) (-15.0379, -3.8523) (-15.0288, -3.8533) (-15.0197, -3.8543) (-15.0106, -3.8553) (-15.0015, -3.8562) (-14.9925, -3.8572) (-14.9835, -3.8581) (-14.9746, -3.859) (-14.9656, -3.8598) (-14.9567, -3.8607) (-14.9479, -3.8615) (-14.939, -3.8624) (-14.9302, -3.8632) (-14.9214, -3.8639) (-14.9127, -3.8647) (-14.9039, -3.8655) (-14.8952, -3.8662) (-14.8866, -3.8669) (-14.8779, -3.8676) (-14.8693, -3.8683) (-14.8608, -3.869) (-14.8522, -3.8696) (-14.8437, -3.8702) (-14.8352, -3.8708) (-14.8268, -3.8714) (-14.8184, -3.872) (-14.81, -3.8726) (-14.8016, -3.8731) (-14.7933, -3.8737) (-14.785, -3.8742) (-14.7768, -3.8747) (-14.7685, -3.8751) (-14.7603, -3.8756) (-14.7522, -3.8761) (-14.744, -3.8765) (-14.7359, -3.8769) (-14.7279, -3.8773) (-14.7199, -3.8777) (-14.7119, -3.878) (-14.7039, -3.8784) (-14.696, -3.8787) (-14.6881, -3.8791) (-14.6802, -3.8794) (-14.6724, -3.8797) (-14.6646, -3.8799) (-14.6568, -3.8802) (-14.6491, -3.8804) (-14.6414, -3.8807) (-14.6338, -3.8809) (-14.6261, -3.8811) (-14.6186, -3.8813) (-14.611, -3.8814) (-14.6035, -3.8816) (-14.596, -3.8817) (-14.5886, -3.8819) (-14.5812, -3.882) (-14.5738, -3.8821) (-14.5665, -3.8822) (-14.5592, -3.8823) (-14.5519, -3.8823) (-14.5447, -3.8824) (-14.5375, -3.8824) (-14.5304, -3.8824) (-14.5233, -3.8824) (-14.5162, -3.8824) (-14.5091, -3.8824) (-14.5021, -3.8824) (-14.4952, -3.8823) (-14.4883, -3.8823) (-14.4814, -3.8822) (-14.4745, -3.8821) (-14.4677, -3.882) (-14.461, -3.8819) (-14.4542, -3.8818) (-14.4476, -3.8817) (-14.4409, -3.8816) (-14.4343, -3.8814) (-14.4277, -3.8812) (-14.4212, -3.8811) (-14.4147, -3.8809) (-14.4083, -3.8807) (-14.4019, -3.8805) (-14.3955, -3.8803) (-14.3892, -3.88) (-14.3829, -3.8798) (-14.3767, -3.8796) (-14.3705, -3.8793) (-14.3643, -3.879) (-14.3582, -3.8788) (-14.3521, -3.8785) (-14.3461, -3.8782) (-14.3401, -3.8779) (-14.3342, -3.8776) (-14.3283, -3.8772) (-14.3224, -3.8769) (-14.3166, -3.8766) (-14.3108, -3.8762) (-14.3051, -3.8758) (-14.2994, -3.8755) (-14.2938, -3.8751) (-14.2882, -3.8747) (-14.2826, -3.8743) (-14.2771, -3.8739) (-14.2717, -3.8735) (-14.2663, -3.8731) (-14.2609, -3.8727) (-14.2556, -3.8723) (-14.2503, -3.8718) (-14.2451, -3.8714) (-14.2399, -3.871) (-14.2348, -3.8705) (-14.2297, -3.87) (-14.2247, -3.8696) (-14.2197, -3.8691) (-14.2148, -3.8686) (-14.2099, -3.8682) (-14.2051, -3.8677) (-14.2003, -3.8672) (-14.1955, -3.8667) (-14.1908, -3.8662) (-14.1862, -3.8657) (-14.1816, -3.8652) (-14.1771, -3.8647) (-14.1726, -3.8642) (-14.1682, -3.8636) (-14.1638, -3.8631) (-14.1594, -3.8626) (-14.1552, -3.8621) (-14.1509, -3.8615) (-14.1467, -3.861) (-14.1426, -3.8605) (-14.1386, -3.86) (-14.1345, -3.8594) (-14.1306, -3.8589) (-14.1267, -3.8583) (-14.1228, -3.8578) (-14.119, -3.8573) (-14.1153, -3.8567) (-14.1116, -3.8562) (-14.1079, -3.8557) (-14.1044, -3.8551) (-14.1009, -3.8546) (-14.0974, -3.854) (-14.094, -3.8535) (-14.0906, -3.853) (-14.0873, -3.8525) (-14.0841, -3.8519) (-14.0809, -3.8514) (-14.0778, -3.8509) (-14.0748, -3.8504) (-14.0718, -3.8498) (-14.0688, -3.8493) (-14.066, -3.8488) (-14.0632, -3.8483) (-14.0604, -3.8478) (-14.0577, -3.8473) (-14.0551, -3.8469) (-14.0525, -3.8464) (-14.05, -3.8459) (-14.0476, -3.8454) (-14.0452, -3.845) (-14.0429, -3.8445) (-14.0407, -3.8441) (-14.0385, -3.8436) (-14.0364, -3.8432) (-14.0343, -3.8428) (-14.0324, -3.8424) (-14.0305, -3.842) (-14.0286, -3.8416) (-14.0268, -3.8412) (-14.0251, -3.8408) (-14.0235, -3.8405) (-14.0219, -3.8401) (-14.0204, -3.8398) (-14.019, -3.8394) (-14.0177, -3.8391) (-14.0164, -3.8388) (-14.0152, -3.8386) (-14.0141, -3.8383) (-14.013, -3.838) (-14.012, -3.8378) (-14.0111, -3.8376) (-14.0103, -3.8374) (-14.0095, -3.8372) (-14.0089, -3.837) (-14.0083, -3.8369) (-14.0077, -3.8367) (-14.0074, -3.8366) (-14.0072, -3.8366) (-14.007, -3.8365) (-14.007, -3.8365) knots -1 -1 -1 -1 -1 -1 -0.99583333 -0.99166667 -0.9875 -0.98333333 -0.97916667 -0.975 -0.97083333 -0.96666667 -0.9625 -0.95833333 -0.95416667 -0.95 -0.94583333 -0.94166667 -0.9375 -0.93333333 -0.92916667 -0.925 -0.92083333 -0.91666667 -0.9125 -0.90833333 -0.90416667 -0.9 -0.89583333 -0.89166667 -0.8875 -0.88333333 -0.87916667 -0.875 -0.87083333 -0.86666667 -0.8625 -0.85833333 -0.85416667 -0.85 -0.84583333 -0.84166667 -0.8375 -0.83333333 -0.82916667 -0.825 -0.82083333 -0.81666667 -0.8125 -0.80833333 -0.80416667 -0.8 -0.79583333 -0.79166667 -0.7875 -0.78333333 -0.77916667 -0.775 -0.77083333 -0.76666667 -0.7625 -0.75833333 -0.75416667 -0.75 -0.74583333 -0.74166667 -0.7375 -0.73333333 -0.72916667 -0.725 -0.72083333 -0.71666667 -0.7125 -0.70833333 -0.70416667 -0.7 -0.69583333 -0.69166667 -0.6875 -0.68333333 -0.67916667 -0.675 -0.67083333 -0.66666667 -0.6625 -0.65833333 -0.65416667 -0.65 -0.64583333 -0.64166667 -0.6375 -0.63333333 -0.62916667 -0.625 -0.62083333 -0.61666667 -0.6125 -0.60833333 -0.60416667 -0.6 -0.59583333 -0.59166667 -0.5875 -0.58333333 -0.57916667 -0.575 -0.57083333 -0.56666667 -0.5625 -0.55833333 -0.55416667 -0.55 -0.54583333 -0.54166667 -0.5375 -0.53333333 -0.52916667 -0.525 -0.52083333 -0.51666667 -0.5125 -0.50833333 -0.50416667 -0.5 -0.49583333 -0.49166667 -0.4875 -0.48333333 -0.47916667 -0.475 -0.47083333 -0.46666667 -0.4625 -0.45833333 -0.45416667 -0.45 -0.44583333 -0.44166667 -0.4375 -0.43333333 -0.42916667 -0.425 -0.42083333 -0.41666667 -0.4125 -0.40833333 -0.40416667 -0.4 -0.39583333 -0.39166667 -0.3875 -0.38333333 -0.37916667 -0.375 -0.37083333 -0.36666667 -0.3625 -0.35833333 -0.35416667 -0.35 -0.34583333 -0.34166667 -0.3375 -0.33333333 -0.32916667 -0.325 -0.32083333 -0.31666667 -0.3125 -0.30833333 -0.30416667 -0.3 -0.29583333 -0.29166667 -0.2875 -0.28333333 -0.27916667 -0.275 -0.27083333 -0.26666667 -0.2625 -0.25833333 -0.25416667 -0.25 -0.24583333 -0.24166667 -0.2375 -0.23333333 -0.22916667 -0.225 -0.22083333 -0.21666667 -0.2125 -0.20833333 -0.20416667 -0.2 -0.19583333 -0.19166667 -0.1875 -0.18333333 -0.17916667 -0.175 -0.17083333 -0.16666667 -0.1625 -0.15833333 -0.15416667 -0.15 -0.14583333 -0.14166667 -0.1375 -0.13333333 -0.12916667 -0.125 -0.12083333 -0.11666667 -0.1125 -0.10833333 -0.10416667 -0.1 -0.09583333 -0.09166667 -0.0875 -0.08333333 -0.07916667 -0.075 -0.07083333 -0.06666667 -0.0625 -0.05833333 -0.05416667 -0.05 -0.04583333 -0.04166667 -0.0375 -0.03333333 -0.02916667 -0.025 -0.02083333 -0.01666667 -0.0125 -0.00833333 -0.00416667 0 0 0 0 0 0
  line L6 (-14.007, -3.8365) -> (-14.0063, -3.8363)
  line L7 (-14.0063, -3.8363) -> (-13.2615, -3.6324)
  arc A4 (-13.2615, -3.6324) -> (-12.8639, -4.8563) centre (0, 0) ccw
  line L8 (-12.8639, -4.8563) -> (-13.5863, -5.129)
  line L9 (-13.5863, -5.129) -> (-13.5869, -5.1293)